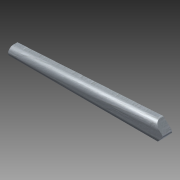
# Autodesk Inventor part: Thrust_Support
Saved by Autodesk Inventor 2011 SP1 (Build 150282100, 282)
## iProperties
Created: 2011-06-11
Part Number: Thrust_Support
Document SubType Name: Modeling
Designer: Andrew G. Meyer
Mass: 5.3795 g
Surface Area: 29.3716 cm^2
Volume: 5.3795 cm^3
Density: 1 g/cm^3
Author: Andrew G. Meyer
Autodesk Inventor part; units mm, degrees
ref_plane "YZ Plane" through (0, 0, 0) normal (1, 0, 0) x (0, 1, 0)
ref_plane "XZ Plane" through (0, 0, 0) normal (0, 1, 0) x (-1, 0, 0)
ref_plane "XY Plane" through (0, 0, 0) normal (0, 0, 1) x (1, 0, 0)
sketch "Sketch1" plane through (0, 0, 0) normal (0, 0, 1) x (1, 0, 0)
  line L0 (-0.7124, 0.6699) -> (-6.35, 5.9705)
  line L1 (-6.35, 5.9705) -> (-103.1875, 0)
  line L2 (-102.9919, -6.35) -> (-5.9705, -6.35)
  line L3 (-5.9705, -6.35) -> (-0.6699, -0.7124)
  arc A0 (-103.1875, 0) -> (-102.9919, -6.35) centre (0, 0) ccw
  arc A1 (-0.7124, 0.6699) -> (-0.6699, -0.7124) centre (0, 0) ccw
  line L4 (0, 0) -> (-0.7124, 0.6699) construction
  line L5 (0, 0) -> (-0.6699, -0.7124) construction
  dimension "d0" = 103.1875
  dimension "d1" = 6.35
  dimension "d2" = 103.1875
  dimension "d3" = 6.35
  dimension "d7" = 1.9558
  constraints: 12 end point, 4 point on circle, 3 perpendicular, 2 centre point, 2 coincident, 2 equal length
  measures "d0" radius of A0
  measures "d1" horizontal distance of point (0, 0) L0.end
  measures "d2" distance of L1.end point (0, 0)
  measures "d3" vertical distance of L2.start L1.end
  measures "d7" diameter of A1
extrude "Extrusion1" add sketch "Sketch1" along normal blind 6.35
fillet "Fillet2" radius 3.81 2 edges at (-54.4812, -6.35, 6.35) (-54.7687, 2.9853, 6.35)
body "Solid1"
